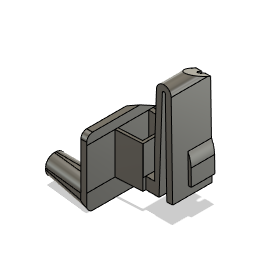
milan-cooler-stuff v10 (Autodesk Fusion 360 design; units mm, degrees)
Autodesk Fusion 360 part; units mm, degrees
note: some values were not read from the file. Chosen so that the rebuilt part matches the saved one: a direction; which face or edge a step refers to.
sketch "Sketch1" plane through (0, 0, 0) normal (0, 0, 1) x (1, 0, 0)
  line L0 (-9.5, -13) -> (-11.5, -13)
  line L1 (-11.5, -13) -> (-11.5, 10)
  line L2 (-11.5, 10) -> (-9.5, 10)
  line L3 (-9.5, 10) -> (-9.5, -13)
  line L4 (-11.5, -13) -> (-11.5, -5) construction
  line L5 (-11.5, -5) -> (-25, -5)
  line L6 (-25, -5) -> (-25, -11.5)
  line L7 (-25, -11.5) -> (-11.5, -13)
  line L8 (-9.5, 7) -> (0, 7)
  line L9 (-9.5, -7) -> (0, -7)
  line L10 (0, 7) -> (0, -7)
  line L11 (0, -7) -> (4, -7)
  line L12 (0, 7) -> (4.5, 7)
  line L13 (4, -7) -> (5.1243, 24.4799)
  line L14 (4.5, 7) -> (2.5013, 7.0714)
  line L15 (4, -7) -> (2, -7)
  line L16 (4, -7) -> (2, -7) construction
  line L17 (2, -7) -> (3.125, 24.5)
  line L18 (3.125, 24.5) -> (8.1247, 24.4498) construction
  line L19 (5.6249, 24.4749) -> (5.5747, 19.4752) construction
  line L20 (6.6176, -7.0263) -> (6.1255, 24.4699)
  line L21 (8.616, -6.9951) -> (8.1247, 24.4498)
  arc A0 (8.1247, 24.4498) -> (3.125, 24.5) centre (5.6249, 24.4749) ccw
  arc A1 (6.1255, 24.4699) -> (5.1243, 24.4799) centre (5.6249, 24.4749) ccw
  line L22 (8.5692, -3.9954) -> (9.569, -3.9798)
  line L23 (8.413, 6.0034) -> (9.4128, 6.019)
  line L24 (9.4128, 6.019) -> (9.569, -3.9798)
  line L25 (6.6176, -7.0263) -> (8.616, -6.9951)
  dimension "d7" = 2
  dimension "d8" = 8
  dimension "d9" = 6.5
  dimension "d10" = 15.5
  dimension "d11" = 9.5
  dimension "d12" = 9.5
  dimension "d13" = 14
  dimension "d14" = 3
  dimension "d15" = 4
  dimension "d16" = 4.5
  dimension "d17" = 31.5
  dimension "d18" = 2
  dimension "d21" = 31.5
  dimension "d23" = 5
  dimension "d24" = 5
  dimension "d25" = 5
  dimension "d26" = 1
  dimension "d27" = 1
  dimension "d29" = 3
  dimension "d30" = 10
  constraint horizontal L0
  constraint vertical L1
  constraint horizontal L2
  constraint vertical L3
  constraint perpendicular L0 L4
  constraint perpendicular L4 L5
  constraint perpendicular L5 L6
  constraint horizontal L8
  constraint coincident L3 L8.start
  constraint coincident L3 L9.start
  constraint perpendicular L3 L9
  constraint perpendicular L10 L11
  constraint perpendicular L10 L12
  constraint perpendicular L13 L14
  constraint midpoint L11 L15.end
  constraint perpendicular L14 L17
  constraint midpoint L18 L19.start
  constraint concentric A0 A1
  constraint coincident L19.start A0.centre
  constraint perpendicular L18 L19
  constraint symmetric L11.end L19 L20.start
  constraint symmetric L13.end L19 L20.end
  constraint symmetric L17.end L19 L18.end
  constraint coincident L21 L22.start
  constraint perpendicular L21 L22
  constraint coincident L21 L23.start
  constraint perpendicular L21 L23
  constraint perpendicular L22 L24
  constraint perpendicular L21 L25
  measures "d7" distance of L0.start L0.end
  measures "d8" distance of L0.end L4.end
  measures "d9" distance of L5.end L6.end
  measures "d10" distance of L3 L6
  measures "d11" distance of L8.start L8.end
  measures "d12" distance of L9.start L9.end
  measures "d13" distance of L8.end L9.end
  measures "d14" distance of L2 L8
  measures "d15" distance of L9.end L11.end
  measures "d16" distance of L8.end L12.end
  measures "d17" distance of L11.end L13.end
  measures "d18" distance of L12.end L14.end
  measures "d21" vertical distance of L15.end L17.end
  measures "d23" distance of L17.end L18.end
  measures "d24" diameter of A0
  measures "d25" distance of L19.start L19.end
  measures "d26" distance of L22.start L22.end
  measures "d27" distance of L23.start L23.end
  measures "d29" distance of L22 L25
  measures "d30" distance of L22 L23
extrude "Extrude1" add sketch "Sketch1" along normal blind 24.5 makes body 1
ref_plane "WorkPlane1" through (0, 28, 0) normal (0, 1, 0) x (0, 0, 1)
sketch "Sketch2" plane through (0, 28, 0) normal (0, 1, 0) x (1, 0, 0)
  line L0 (-11.4956, -24.5039) -> (-11.4956, -16.5039)
  line L1 (-11.4956, -16.5039) -> (-24.9956, -16.5039)
  line L2 (-24.9956, -16.5039) -> (-24.9956, -23.0039)
  line L3 (-24.9956, -23.0039) -> (-11.4956, -24.5039)
  line L4 (-11.4956, -16.5039) -> (-9, -16.5039) construction
  line L5 (-11.4956, -24.5039) -> (-9.4956, -24.5039)
  line L6 (-11.4956, -0.0039) -> (-11.4956, -16.5039)
  line L7 (-9.4956, -24.5039) -> (-9.4956, -15)
  line L8 (-11.4956, -0.0039) -> (-9.4956, -0.0039)
  line L9 (-9.4956, -0.0039) -> (-9.4956, -1.9039)
  line L10 (-9.4956, -1.9039) -> (-9.4956, -14.9039)
  line L11 (-9.4956, -14.9039) -> (-9.4956, -15)
  line L12 (-9.4956, -8.4039) -> (-0.4956, -8.4039) construction
  line L13 (-0.4956, -8.4039) -> (-0.4956, -2.4039) construction
  line L14 (-0.4956, -8.4039) -> (-0.4956, -14.4039) construction
  line L15 (-9.4956, -14.9039) -> (-0.4956, -14.4039)
  line L16 (-9.4956, -1.9039) -> (-0.4956, -2.4039)
  line L17 (-0.4956, -2.4039) -> (-0.4956, -14.4039)
  line L18 (-9.4956, -13.9024) -> (-1.4956, -13.4579)
  line L19 (-9.4956, -3.4062) -> (-1.4956, -3.8507)
  line L20 (-1.4956, -3.8507) -> (-1.4956, -13.4579)
  circle A0 centre (-0.4956, -14.4039) radius 1 construction
  line L21 (-0.4956, -13.4039) -> (11.5044, -13.4039)
  line L22 (-0.4956, -2.4039) -> (2.0044, -2.4039)
  line L23 (2.0044, -2.4039) -> (2.0044, 1.5961)
  line L24 (2.0044, 1.5961) -> (11.5044, 1.5961)
  line L25 (11.5044, -13.4039) -> (11.5044, 1.5961)
  dimension "d34" = 8
  dimension "d35" = 6.5
  dimension "d37" = 2
  dimension "d68" = 15.5
  dimension "d95" = 1.9
  dimension "d96" = 13
  dimension "d97" = 24.5
  dimension "d98" = 9
  dimension "d100" = 6
  dimension "d101" = 6
  dimension "d102" = 1.5
  dimension "d103" = 1
  dimension "d104" = 1
  dimension "d105" = 2
  dimension "d106" = 12
  dimension "d107" = 2.5
  dimension "d108" = 4
  constraint vertical L0
  constraint perpendicular L0 L1
  constraint perpendicular L1 L2
  constraint perpendicular L0 L4
  constraint perpendicular L0 L5
  constraint perpendicular L1 L6
  constraint perpendicular L6 L8
  constraint perpendicular L8 L9
  constraint parallel L7 L10
  constraint parallel L7 L11
  constraint midpoint L10 L12.start
  constraint perpendicular L10 L12
  constraint vertical L13
  constraint vertical L14
  constraint parallel L16 L19
  constraint parallel L15 L18
  constraint vertical L20
  constraint coincident L10 L19.start
  constraint coincident L10 L18.start
  constraint coincident L14.end L15.end
  constraint coincident L17 L21.start
  constraint coincident A0 L21.start
  constraint perpendicular L17 L21
  constraint perpendicular L17 L22
  constraint perpendicular L22 L23
  constraint perpendicular L23 L24
  constraint perpendicular L21 L25
  measures "d34" distance of L0.start L0.end
  measures "d35" distance of L1.end L2.end
  measures "d37" distance of L0.start L5.end
  measures "d68" distance of L2 L7
  measures "d95" distance of L8.end L9.end
  measures "d96" distance of L9.end L10.end
  measures "d97" distance of L5 L8
  measures "d98" distance of L12.start L12.end
  measures "d100" distance of L12.end L13.end
  measures "d101" distance of L12.end L14.end
  measures "d102" distance of L16 L19
  measures "d103" distance of L15 L18
  measures "d104" distance of L14 L20
  measures "d105" diameter of A0
  measures "d106" distance of L21.start L21.end
  measures "d107" distance of L13.end L22.end
  measures "d108" distance of L22.end L23.end
extrude "Extrude2" cut sketch "Sketch2" against normal blind 50 contours L0 L1 L2 L3 | L0 L5 L6 L7 L8 L9 L10 L11 | L10 L15 L16 L17 L18 L19 L20 | L17 L21 L22 L23 L24 L25 keep common part bodies 1
sketch "Sketch3" plane through (0, 0, 13.5) normal (0, 0, 1) x (1, 0, 0)
  line L0 (0, 7) -> (-0.5, 7)
  line L1 (-0.5, 7) -> (-0.5, -7)
  line L2 (-0.5, -7) -> (0, -7)
  line L3 (0, -7) -> (4, -7)
  line L4 (4, -7) -> (5.1243, 24.4799)
  arc A0 (6.1255, 24.4699) -> (5.1243, 24.4799) centre (5.6249, 24.4749) ccw
  line L5 (6.1255, 24.4699) -> (6.6176, -7.0263)
  line L6 (6.6176, -7.0263) -> (8.616, -6.9951)
  line L7 (8.616, -6.9951) -> (8.5692, -3.9954)
  line L8 (8.5692, -3.9954) -> (9.569, -3.9798)
  line L9 (9.569, -3.9798) -> (9.4128, 6.019)
  line L10 (9.4128, 6.019) -> (8.413, 6.0034)
  line L11 (8.413, 6.0034) -> (8.1247, 24.4498)
  arc A1 (8.1247, 24.4498) -> (3.125, 24.5) centre (5.6249, 24.4749) ccw
  line L12 (3.125, 24.5) -> (2.5, 7)
  line L13 (2.5, 7) -> (0, 7)
  line L14 (8.413, 6.0034) -> (8.5692, -3.9954)
  line L15 (9.569, -3.9798) -> (9.4128, 6.019)
  line L16 (8.413, 6.0034) -> (9.4128, 6.019)
  constraint coincident L10.end L11.start
  constraint coincident L7.end L8.start
  constraint coincident L8.end L9.start
  constraint coincident L9.end L10.start
extrude "Extrude3" cut sketch "Sketch3" against normal blind 5.5 contours L8 L9 L10 L14 L15 L16 bodies 1
fillet "Fillet1" radius 10 1 edges at (9.4128, 6.019, 4) on bodies 1
fillet "Fillet2" radius 3 4 edges at (-18.2632, -5, 23.752) (-18.2632, -12.2485, 23.752) (-18.2478, -12.2502, 16.5039) (-18.2478, -5, 16.5039) on bodies 1
fillet "Fillet3" radius 2 1 edges at (-10.5, 10, 24.5) on bodies 1
ref_plane "WorkPlane2" through (10, 0, 0) normal (1, 0, 0) x (0, 1, 0)
sketch "Sketch4" plane through (10, 0, 0) normal (1, 0, 0) x (0, 0, -1)
  line L0 (0, 24) -> (-6.5, 27)
  line L1 (-6.5, 27) -> (0, 27)
  line L2 (0, 27) -> (0, 24)
extrude "Extrude4" cut sketch "Sketch4" against normal blind 14 bodies 1
ref_plane "WorkPlane3" through (0, 7, 0) normal (0, 1, 0) x (0, 0, 1)
sketch "Sketch7" plane through (0, 7, 0) normal (0, 1, 0) x (1, 0, 0)
  line L0 (-0.5, 0.2561) -> (-0.5, -7) construction
  line L1 (-0.5, -7) -> (2.5, -7)
  line L2 (2.5, -7) -> (2.5, -9)
  line L3 (2.5, -9) -> (-0.5, -9)
  line L4 (-0.5, -9) -> (-0.5, -13) construction
  line L5 (-0.5, -7) -> (-0.5, -9)
  line L6 (-0.5, 0.2561) -> (2.5, 0.2561)
  line L7 (2.5, 0.2561) -> (2.5, -7)
  line L8 (2.5, -7) -> (-0.5, -7)
  line L9 (-0.5, -7) -> (-0.5, 0.2561)
  line L10 (-0.5, -9) -> (2.5, -9)
  line L11 (2.5, -9) -> (2.5, -14.2665)
  line L12 (2.5, -14.2665) -> (-0.5, -14.2665)
  line L13 (-0.5, -14.2665) -> (-0.5, -9)
  dimension "d109" = 2
  dimension "d114" = 3
  constraint vertical L0
  constraint perpendicular L0 L1
  constraint perpendicular L1 L2
  constraint perpendicular L0 L3
  constraint perpendicular L3 L4
  constraint perpendicular L3 L5
  constraint horizontal L6
  constraint vertical L7
  constraint horizontal L8
  constraint vertical L9
  constraint horizontal L10
  constraint vertical L11
  constraint horizontal L12
  constraint vertical L13
  measures "d109" distance of L1.end L2.end
  measures "d114" distance of L7 L9
extrude "Extrude6" cut sketch "Sketch7" against normal blind 1.5 bodies 1
extrude "Extrude7" cut sketch "Sketch7" against normal blind 10 contours L1 L6 L7 L8 L9 | L3 L10 L11 L12 L13 bodies 1
sketch "Sketch8" plane through (0, -3, 0) normal (0, 1, 0) x (-1, 0, 0)
  line L0 (-2.5, 0) -> (-2.0044, 0)
  line L1 (-2.0044, 0) -> (-2.0044, 2.4039)
  line L2 (-2.0044, 2.4039) -> (0.4956, 2.4039)
  line L3 (0.4956, 2.4039) -> (0.5, 2.4037)
  line L4 (0.5, 2.4037) -> (0.5, 7)
  line L5 (0.5, 7) -> (-2.5, 7)
  line L6 (-2.5, 7) -> (-2.5, 0)
  line L7 (-2.0044, 0) -> (-2.5, 0)
  line L8 (-2.5, 0) -> (-2.5, 2.3977)
  line L9 (-2.5, 2.3977) -> (-2.0044, 2.3977)
  line L10 (-2.0044, 2.3977) -> (-2.0044, 0)
  constraint horizontal L7
  constraint vertical L8
  constraint horizontal L9
  constraint vertical L10
  constraint coincident L6 L8.end
  constraint coincident L0.end L1.start
extrude "Extrude8" cut sketch "Sketch8" against normal blind 5.2 contours L0 L1 L6 L7 L8 L9 L10 bodies 1
ref_plane "WorkPlane4" through (0, 10.5, 0) normal (0, 1, 0) x (0, 0, 1)
sketch "Sketch9" plane through (0, 10.5, 0) normal (0, 1, 0) x (1, 0, 0)
  line L0 (3.5, -6.5) -> (7.5, -6.5)
  line L1 (7.5, -6.5) -> (7.5, -7.5)
  line L2 (7.5, -7.5) -> (3.5, -7.5)
  line L3 (3.5, -7.5) -> (3.5, -6.5)
  dimension "d118" = 1
  constraint horizontal L0
  constraint vertical L1
  constraint horizontal L2
  constraint vertical L3
  measures "d118" distance of L0.start L2.end
extrude "Extrude9" add sketch "Sketch9" along normal blind 15 separate body makes body 2
combine "Combine1" operation add target body 1 tool bodies 2 keep tools
sketch "Sketch10" plane through (-11.4956, 0, 0) normal (-1, 0, 0) x (0, 0, 1)
  line L0 (0.0039, -13) -> (19.45, -13)
  ellipse E0 centre (19.5039, -9.982) end of major axis (19.5039, -13.0005) minor radius 3 (16.5039, -9.982) -> (19.45, -13) ccw
  line L1 (16.5039, -9.982) -> (16.5039, 10)
  line L2 (16.5039, 10) -> (0.0039, 10)
  line L3 (0.0039, 10) -> (0.0039, -13)
  line L4 (0.0039, 10) -> (9.0039, 10)
  line L5 (9.0039, 10) -> (9.0039, 6)
  line L6 (9.0039, 6, 0) -> (0.0039, 6.7234, -2.2943)
  line L7 (0.0039, 6.7234, -2.2943) -> (0.0039, 10, 0)
  line L8 (9.0039, 10, 0) -> (0.0039, 6.7234, -2.2943)
  dimension "d124" = 9
  dimension "d125" = 4
  constraint coincident L2.end L3.start
  measures "d124" distance of L2.end L4.end
sketch "Sketch10 (curves on the plane with normal -0.8192, -0.5736, 0 at -5.7358 mm)" plane through (-6.7972, 3.2899, 0) normal (-0.819152, -0.573576, 0) x (0, 0, 1)
  line L0 (16.5039, 8.1915) -> (0.0039, 8.1915)
  line L1 (0.0039, 8.1915) -> (9.0039, 8.1915)
  line L2 (0.0039, 4.1915) -> (0.0039, 8.1915)
  line L3 (9.0039, 8.1915) -> (0.0039, 4.1915)
extrude "Extrude10" cut sketch "Sketch10 (curves on the plane with normal -0.8192, -0.5736, 0 at -5.7358 mm)" along normal mid plane 9 bodies 1
hidden bodies 2
